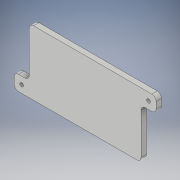
# Autodesk Inventor part: Дно Модуля БП
Saved by Autodesk Inventor 2019 (Build 230136000, 136)
## iProperties
Created: 2018-07-03
Part Number: Дно Модуля БП
Material: Типовые
Document SubType Name: Modeling
Designer: rossolov
Density: 1 g/cm^3
Appearance: По умолчанию
Author: rossolov
Autodesk Inventor part; units mm, degrees
ref_plane "YZ Plane" through (0, 0, 0) normal (1, 0, 0) x (0, 1, 0)
ref_plane "XZ Plane" through (0, 0, 0) normal (0, 1, 0) x (-1, 0, 0)
ref_plane "XY Plane" through (0, 0, 0) normal (0, 0, 1) x (1, 0, 0)
sketch "Эскиз1" plane through (0, 0, 0) normal (0, 0, 1) x (1, 0, 0)
  line L0 (-21.8917, 12.7106) -> (30.1083, 12.7106)
  line L1 (30.1083, 5.7106) -> (30.1083, -17.2894)
  line L2 (30.1083, -17.2894) -> (-21.8917, -17.2894)
  line L3 (-21.8917, -10.2894) -> (-21.8917, 12.7106)
  line L4 (-21.8917, -17.2894) -> (-28.8917, -17.2894)
  line L5 (-28.8917, -17.2894) -> (-28.8917, -10.2894)
  line L6 (-28.8917, -10.2894) -> (-21.8917, -10.2894)
  line L7 (30.1083, 12.7106) -> (37.1083, 12.7106)
  line L8 (37.1083, 12.7106) -> (37.1083, 5.7106)
  line L9 (37.1083, 5.7106) -> (30.1083, 5.7106)
  point P0 (0, 0)
  dimension "d3" = 7
  dimension "d5" = 7
  constraints: 20 end point, 4 parallel, 3 horizontal, 3 perpendicular
  measures "d3" distance of L4.end L5.end
  measures "d5" distance of L7.end L8.end
extrude "Выдавливание1" add sketch "Эскиз1" along normal blind 2.5
fillet "Сопряжение1" radius 2 6 edges at (37.1083, 12.7106, 1.25) (37.1083, 5.7106, 1.25) (30.1083, -17.2894, 1.25) (-28.8917, -10.2894, 1.25) (-21.8917, 12.7106, 1.25) (-28.8917, -17.2894, 1.25)
fillet "Сопряжение2" radius 2 2 edges at (-21.8917, -10.2894, 1.25) (30.1083, 5.7106, 1.25)
sketch "Эскиз2" plane through (0, 0, 2.5) normal (0, 0, 1) x (1, 0, 0)
  arc A0 (-26.8917, -10.2894) -> (-28.8917, -12.2894) centre (-26.8917, -12.2894) ccw projected
  circle A1 centre (-25.3917, -13.7894) radius 0.85
  circle A2 centre (33.6083, 9.2106) radius 0.85
  point P0 (0, 0)
  point P1 (37.1083, 10.7106)
  point P2 (35.1083, 5.7106)
  dimension "d12" = 1.7
  dimension "d15" = 1.7
  constraints: 2 centre point
  measures "d12" diameter of A1
  measures "d15" diameter of A2
extrude "Выдавливание2" cut sketch "Эскиз2" against normal blind 2.5
sketch "Эскиз3" plane through (0, 0, 0) normal (0, 0, -1) x (-1, 0, 0)
  arc A0 (21.8917, 10.7106) -> (19.8917, 12.7106) centre (19.8917, 10.7106) ccw projected
  line L0 (-28.1083, -17.2894) -> (26.8917, -17.2894) projected
  line L1 (-19.2442, -15.1834) -> (19.7856, -15.1834)
  line L2 (19.7856, -15.1834) -> (19.7856, 3.4434)
  line L3 (10.2125, 10.6045) -> (-28.0023, 10.6045)
  line L4 (-28.0023, 10.6045) -> (-28.0023, -8.0395)
  line L5 (19.7856, -15.1834) -> (22.7856, -15.1834) construction
  line L6 (17.6643, -13.062) -> (-19.2442, -13.062)
  line L7 (-25.8809, -8.0395) -> (-25.8809, 8.4832)
  line L8 (-25.8809, 8.4832) -> (10.2125, 8.4832)
  line L9 (17.6643, 3.4434) -> (17.6643, -13.062)
  line L10 (10.2125, 10.6045) -> (10.2125, 8.4832)
  line L11 (19.7856, 3.4434) -> (17.6643, 3.4434)
  line L12 (-19.2442, -15.1834) -> (-19.2442, -13.062)
  line L13 (-28.0023, -8.0395) -> (-25.8809, -8.0395)
  point P0 (0, 0)
  constraints: 26 end point, 5 perpendicular, 4 horizontal, 4 parallel
extrude "Выдавливание3" add sketch "Эскиз3" along normal blind 2
fillet "Сопряжение3" radius 2 4 edges at (-18.7249, 3.4434, -2) (-10.2125, 9.5438, -2) (26.9416, -8.0395, -2) (19.2442, -14.1227, -2)
